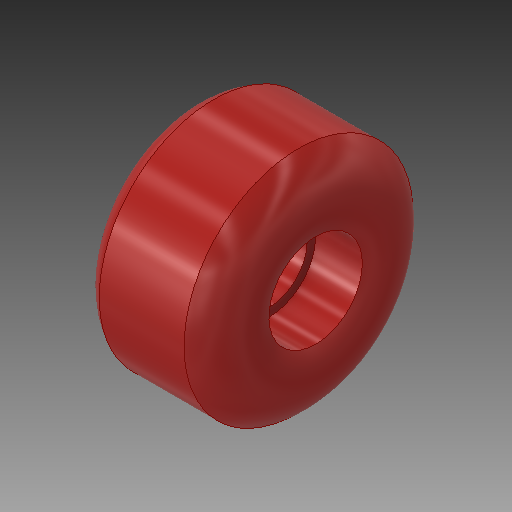
# Autodesk Inventor part: Wheels 54mm cut
Saved by Autodesk Inventor 2019 (Build 230136000, 136)
## iProperties
Created: 2020-12-02
Part Number: Wheels 54mm cut
Material: Generic
Document SubType Name: Modeling
Designer: Anass Hamdi
Density: 1 g/cm^3
Appearance: Orange-Red
Author: Anass Hamdi
Autodesk Inventor part; units mm, degrees
ref_plane "YZ Plane" through (0, 0, 0) normal (1, 0, 0) x (0, 1, 0)
ref_plane "XZ Plane" through (0, 0, 0) normal (0, 1, 0) x (-1, 0, 0)
ref_plane "XY Plane" through (0, 0, 0) normal (0, 0, 1) x (1, 0, 0)
sketch "Sketch1" plane through (0, 0, 0) normal (0, 0, 1) x (1, 0, 0)
  line L0 (0, -27.001) -> (0, -11.001) construction
  line L1 (-10, -27.001) -> (10, -27.001)
  line L2 (-10, -11.001) -> (-3, -11.001)
  line L3 (10, -11.001) -> (10, -27.001) construction
  line L4 (-10, -27.001) -> (-15, -27.001) construction
  line L5 (-15, -27.001) -> (-15, -22.001) construction
  line L6 (-10, -11.001) -> (-13, -11.001)
  arc A0 (-15, -22.001) -> (-10, -27.001) centre (-5.9615, -17.9625) ccw
  line L7 (-13, -11.001) -> (-15, -11.001) construction
  line L8 (-15, -11.001) -> (-15, -13.001) construction
  spline S0 degree 2 poles (-13, -11.001) (-14.3797, -11.3969) (-15, -13.001) knots 0 0 0 1 1 1
  spline S1 degree 4 poles (-15, -13.001) (-14.9648, -13.7958) (-13.1729, -17.7088) (-14.1493, -19.5238) (-15.338, -21.3003) (-15, -22.001) knots 0 0 0 0 0 0.555386 1 1 1 1 1
  line L9 (10, -11.001) -> (14, -11.001)
  line L10 (10, -19.001) -> (15, -19.001) construction
  arc A1 (10, -27.001) -> (14, -11.001) centre (2.1667, -16.5427) ccw
  line L11 (0, 0) -> (0, -11.001) construction
  line L12 (-21.9226, 0) -> (23.3042, 0) projected
  line L13 (0, -11.001) -> (0.5, -11.001) construction
  line L14 (0.5, -11.001) -> (0.5, 0) construction
  line L15 (0.5, -11.001) -> (0.5, -9.001) construction
  line L16 (0.5, -9.001) -> (3, -9.001)
  line L17 (0.5, -9.001) -> (-3, -9.001)
  line L18 (3, -9.001) -> (3, -11.001)
  line L19 (-3, -9.001) -> (-3, -11.001)
  line L20 (0, -11.001) -> (3, -11.001) construction
  line L21 (3, -11.001) -> (10, -11.001)
  line L22 (-3, -11.001) -> (0, -11.001) construction
  point P0 (-14.1392, -11.6496)
  point P1 (-14.4314, -15.1293)
  point P2 (-14.4314, -19.7118)
  point P3 (-15, -21.0187)
  point P4 (-14, -17.9625)
  dimension "d1" = 16
  dimension "d3" = 20
  dimension "d4" = 20
  dimension "d17" = 5
  dimension "d18" = 5
  dimension "d20" = 3
  dimension "d21" = 2
  dimension "d22" = 2
  dimension "d23" = 4
  dimension "d24" = 5
  dimension "d25" = 11.001
  dimension "d26" = 14
  dimension "d28" = 13
  dimension "d29" = 0.5
  dimension "d30" = 2
  dimension "d31" = 2.5
  dimension "d32" = 3.5
  constraints: 44 end point, 11 horizontal, 11 perpendicular, 5 point on circle, 5 point on line, 4 vertical, 2 centre point, 2 midpoint, 9 other
  measures "d1" distance of L0.start L0.end
  measures "d3" distance of L1.start L1.end
  measures "d4" distance of L2.start L3.start
  measures "d17" distance of L1.start L4.end
  measures "d18" distance of L5.end L4.end
  measures "d20" distance of L6.end L2.start
  measures "d21" distance of L6.end L7.end
  measures "d22" distance of L7.end L8.end
  measures "d23" distance of L3.start L9.end
  measures "d24" distance of L10.start L10.end
  measures "d25" distance of L11.start L11.end
  measures "d26" distance from line of L0 L9.end
  measures "d28" distance of L6.end L0.end
  measures "d29" distance of L11.end L13.end
  measures "d30" distance of L13.end L15.end
  measures "d31" distance of L15.end L16.end
  measures "d32" distance of L15.end L17.end
revolve "Revolution1" add sketch "Sketch1" angle 360 about axis through (-10, 0, 0) along (1, 0, 0)
body "Solid1"
